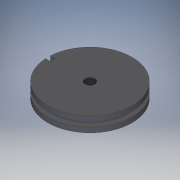
# Autodesk Inventor part: Polia2
Saved by Autodesk Inventor 2018 (Build 220112000, 112)
## iProperties
Created: 2017-05-31
Part Number: Polia2
Material: Genérico
Document SubType Name: Modeling
Designer: Vitor
Density: 1 g/cm^3
Appearance: Padrão
Author: Vitor
Autodesk Inventor part; units mm, degrees
ref_plane "YZ Plane" through (0, 0, 0) normal (1, 0, 0) x (0, 1, 0)
ref_plane "XZ Plane" through (0, 0, 0) normal (0, 1, 0) x (-1, 0, 0)
ref_plane "XY Plane" through (0, 0, 0) normal (0, 0, 1) x (1, 0, 0)
sketch "Esboço1" plane through (0, 0, 0) normal (0, 0, 1) x (1, 0, 0)
  circle A0 centre (0, 0) radius 5
  dimension "d0" = 10
  constraints: 1 centre point, 1 coincident
  measures "d0" diameter of A0
extrude "Extrusão1" add sketch "Esboço1" along normal blind 1
sketch "Esboço2" plane through (0, 0, 1) normal (0, 0, 1) x (1, 0, 0)
  circle A0 centre (0, 0) radius 4
  dimension "d3" = 8
  constraints: 1 centre point, 1 coincident
  measures "d3" diameter of A0
extrude "Extrusão2" add sketch "Esboço2" along normal blind 1
sketch "Esboço3" plane through (0, 0, 2) normal (0, 0, 1) x (1, 0, 0)
  circle A0 centre (0, 0) radius 5
  dimension "d6" = 10
  constraints: 1 centre point, 1 coincident
  measures "d6" diameter of A0
extrude "Extrusão3" add sketch "Esboço3" along normal blind 1
sketch "Esboço4" plane through (0, 0, 3) normal (0, 0, 1) x (1, 0, 0)
  circle A0 centre (0, 0) radius 4 projected
  circle A1 centre (0, 0) radius 1
  dimension "d9" = 2
  constraints: 1 centre point, 1 coincident
  measures "d9" diameter of A1
extrude "Extrusão4" cut sketch "Esboço4" against normal blind 4 contours A1
thread "Rosca1" size "M2x0.4" class "6H" standard "ANSI Metric M Profile" full length
sketch "Esboço5" plane through (0, 0, 3) normal (0, 0, 1) x (1, 0, 0)
  circle A0 centre (0, 0) radius 5 projected
  line L0 (-4, 0) -> (-4, -0.5)
  circle A1 centre (0, 0) radius 4 projected
  line L1 (-4, 0) -> (-3.5, 0) construction
  line L2 (-4, -0.5) -> (-5, -0.5)
  line L3 (-5, -0.5) -> (-5, 0.5)
  line L4 (-5, -0.5) -> (-4, -0.5) construction
  line L5 (-5, 0.5) -> (-4, 0.5)
  line L6 (-4, 0.5) -> (-4, 0)
  line L7 (-4, -0.5) -> (-5, -0.5)
  dimension "d15" = 0.5
  dimension "d16" = 90
  dimension "d17" = 1
  dimension "d18" = 90
  constraints: 16 end point, 6 perpendicular, 3 vertical, 2 horizontal, 1 collinear, 1 horizontal alignment
  measures "d15" distance of L0.start L0.end
  measures "d16" angle of L0 L1
  measures "d17" distance of L2.end L3.end
  measures "d18" angle of L4 L3
extrude "Extrusão5" cut sketch "Esboço5" against normal blind 10 contours L5 L6 L0 L2 A0 | A0 L3 L5 | L2 L3 A0 picked at (-4.3296, -0.2779)
sketch "Esboço7" plane through (0, 0, 3) normal (0, 0, 1) x (1, 0, 0)
  circle A0 centre (0, 0) radius 1 projected
  circle A1 centre (0, 0) radius 1
  circle A2 centre (0, 0) radius 8.5
  line L0 (-8.5, 0) -> (-7.5, 0)
  line L1 (-7.5, 0) -> (-7.5, -0.5)
  line L2 (-7.5, -0.5) -> (-8.4853, -0.5)
  line L3 (-7.5, 0) -> (-7.5, 0.5)
  line L4 (-7.5, 0.5) -> (-8.4853, 0.5)
  dimension "d21" = 17
  dimension "d22" = 1
  dimension "d23" = 0.5
  dimension "d24" = 0.5
  constraints: 10 end point, 3 perpendicular, 3 point on circle, 2 centre point, 2 coincident, 1 horizontal, 1 point on line
  measures "d21" diameter of A2
  measures "d22" distance of L0.start L0.end
  measures "d23" distance of L0.end L1.end
  measures "d24" distance of L0.end L3.end
extrude "Extrusão6" add sketch "Esboço7" against normal blind 1 contours A2 L2 L1 L3 L4
sketch "Esboço8" plane through (0, 0, 2) normal (0, 0, -1) x (-1, 0, 0)
  circle A0 centre (0, 0) radius 1
  circle A1 centre (0, 0) radius 1 projected
  circle A2 centre (0, 0) radius 7.5
  dimension "d27" = 15
  constraints: 2 centre point, 2 coincident
  measures "d27" diameter of A2
extrude "Extrusão7" add sketch "Esboço8" along normal blind 1
sketch "Esboço9" plane through (0, 0, 0) normal (0, 0, -1) x (-1, 0, 0)
  circle A0 centre (0, 0) radius 1
  circle A1 centre (0, 0) radius 8.5
  line L0 (8.4853, -0.5) -> (7.5, -0.5) projected
  line L1 (7.5, 0) -> (7.5, -0.5)
  line L2 (7.5, -0.5) -> (8.4853, -0.5)
  line L3 (8.4853, -0.5) -> (8.4853, 0.5)
  line L4 (8.4853, 0.5) -> (7.5, 0.5) projected
  line L5 (7.5, 0.5) -> (8.4853, 0.5)
  line L6 (7.5, -0.5) -> (7.5, 0.5)
  constraints: 10 end point, 3 collinear, 2 centre point, 2 coincident, 2 perpendicular, 1 point on circle
extrude "Extrusão8" add sketch "Esboço9" against normal blind 1 contours L4 L6 L1 L0 A1
